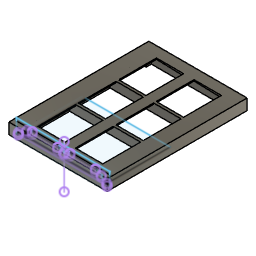
case_basic_v1 (Autodesk Fusion 360 archive; units mm, degrees)
design "lid fitting"
Autodesk Fusion 360 part; units mm, degrees
sketch "Skizze1" plane through (0, 0, 0) normal (0, 1, 0) x (1, 0, 0)
  line L0 (0, 0) -> (66.84, 0)
  line L1 (66.84, 0) -> (66.84, -1.6)
  line L2 (66.84, -1.6) -> (0, -1.6)
  line L3 (0, -1.6) -> (0, 0)
  line L4 (6.12, -13) -> (6.12, 20) construction
  line L5 (6.12, -4.35) -> (34.0577, -3.52)
  line L6 (6.1556, -5.5495) -> (34.0933, -4.7195)
  line L7 (34.0933, -4.7195) -> (34.0577, -3.52)
  line L8 (6.1556, -5.5495) -> (6.12, -4.35)
  line L9 (10.5057, -7.171) -> (29.6972, -6.6008)
  line L10 (10.5057, -7.171) -> (10.4537, -5.4218)
  line L11 (29.6972, -6.6008) -> (29.6453, -4.8516)
  line L12 (34.6056, -5.5495) -> (62.5433, -4.7195)
  line L13 (34.57, -13) -> (34.57, 20) construction
  line L14 (38.9557, -7.171) -> (38.9037, -5.4218)
  line L15 (34.57, -4.35) -> (62.5077, -3.52)
  line L16 (34.6056, -5.5495) -> (34.57, -4.35)
  line L17 (38.9557, -7.171) -> (58.1472, -6.6008)
  line L18 (62.5433, -4.7195) -> (62.5077, -3.52)
  line L19 (58.1472, -6.6008) -> (58.0953, -4.8516)
  dimension "d1" = 66.84
  dimension "d2" = 1.6
  dimension "d3" = 6.12
  dimension "d4" = 2.75
  dimension "d5" = 1.92
  dimension "d6" = 27.95
  dimension "d7" = 1.2
  dimension "d8" = 1.75
  dimension "d9" = 4.3
  dimension "d10" = 19.2
  dimension "d11" = 1.2
  dimension "d12" = 27.95
  dimension "d13" = 1.75
  dimension "d14" = 4.3
  dimension "d15" = 19.2
  constraint horizontal L0
  constraint vertical L1
  constraint horizontal L2
  constraint vertical L3
  constraint coincident L0.start L3.end
  constraint perpendicular L0 L4
  constraint coincident L4 L5.start
  constraint perpendicular L5 L7
  constraint perpendicular L5 L8
  constraint parallel L6 L9
  constraint coincident L6 L10.end
  constraint perpendicular L6 L10
  constraint coincident L6 L11.end
  constraint perpendicular L6 L11
  constraint coincident L15.start L13
  constraint perpendicular L15 L18
  constraint perpendicular L15 L16
  constraint parallel L12 L17
  constraint coincident L14.end L12
  constraint perpendicular L12 L14
  constraint coincident L19.end L12
  constraint perpendicular L12 L19
  measures "d1" distance of L0.start L0.end
  measures "d2" distance of L0.start L2.end
  measures "d3" distance of L3 L4
  measures "d4" distance of L2 L5.start
  measures "d5" distance of L2 L5.end
  measures "d6" distance of L5.start L5.end
  measures "d8" distance of L6 L9
  measures "d9" distance of L8 L10
  measures "d10" distance of L10 L11
  measures "d12" distance of L15.end L15.start
  measures "d13" distance of L12 L17
  measures "d14" distance of L14 L16
  measures "d15" distance of L14 L19
sketch "Skizze2" plane through (0, 0, 0) normal (0, 1, 0) x (1, 0, 0)
  line L0 (0, -1.65) -> (5.6396, -1.65)
  line L1 (5.6396, -1.65) -> (5.8137, -7.5105)
  line L2 (5.8137, -7.5105) -> (30.6972, -6.7712)
  line L3 (34.5575, -5.9701) -> (34.6029, -7.5004)
  line L4 (34.6029, -7.5004) -> (59.1472, -6.7712)
  line L5 (63.4939, -1.65) -> (67.24, -1.65)
  line L6 (67.24, -1.65) -> (67.24, 0)
  line L7 (0, -1.65) -> (-0.4, -1.65)
  line L8 (-0.4, -1.65) -> (-0.4, 0)
  line L9 (-0.4, 0) -> (-1.5, 0)
  line L10 (-1.5, 0) -> (-1.5, -10.4859)
  line L11 (-1.5, -10.4859) -> (69, -10.4859)
  line L12 (69, -10.4859) -> (69, 0)
  line L13 (69, 0) -> (67.24, 0)
  line L14 (10.5057, -7.171) -> (29.6972, -6.6008)
  line L15 (38.9557, -7.171) -> (58.1472, -6.6008)
  line L16 (38.9557, -7.171) -> (38.9037, -5.4218)
  line L17 (34.6056, -5.5495) -> (62.5433, -4.7195)
  line L18 (34.6056, -5.5495) -> (34.57, -4.35)
  line L19 (6.1556, -5.5495) -> (34.0933, -4.7195)
  line L20 (29.6972, -6.6008) -> (29.6453, -4.8516)
  line L21 (6.1556, -5.5495) -> (6.12, -4.35)
  line L22 (62.5433, -4.7195) -> (62.5077, -3.52)
  line L23 (58.1472, -6.6008) -> (58.0953, -4.8516)
  line L24 (0, -1.6) -> (0, 0)
  line L25 (66.84, -1.6) -> (0, -1.6)
  line L26 (10.5057, -7.171) -> (10.4537, -5.4218)
  line L27 (66.84, 0) -> (66.84, -1.6)
  line L28 (59.1472, -6.7712) -> (63.3193, -5.3134)
  line L29 (30.6972, -6.7712) -> (34.5575, -5.9701)
  line L30 (34.6029, -7.5004) -> (30.6972, -8.2712)
  line L31 (30.6972, -8.2712) -> (30.6972, -6.7712)
  line L32 (34.57, -13) -> (34.57, 20)
  line L33 (59.1472, -6.7712) -> (59.1472, -8.2712)
  line L34 (59.1472, -8.2712) -> (69, -8.2712)
  line L35 (30.6972, -8.2712) -> (38.5, -8.2712)
  line L36 (38.5, -8.2712) -> (38.5, -7.3846)
  line L37 (10.1496, -8.2712) -> (10.1496, -7.3817)
  line L38 (10.1496, -8.2712) -> (6, -8.2712)
  line L39 (6, -8.2712) -> (-1.5, -8.2712)
  line L40 (10.1496, -8.2712) -> (30.6972, -8.2712)
  line L41 (38.5, -8.2712) -> (59.1472, -8.2712)
  line L42 (0, 0) -> (66.84, 0)
  line L43 (-0.4, -1.65) -> (67.24, -1.65)
  line L44 (-0.4, 0) -> (67.24, 0)
  line L45 (63.3193, -5.3134) -> (63.4939, -1.65)
  dimension "d16" = 0.4
  dimension "d17" = 0.05
  dimension "d18" = 0.4
  dimension "d21" = 0.2
  dimension "d27" = 0.2
  dimension "d32" = 0.05
  dimension "d33" = 0.4
  dimension "d39" = 1
  dimension "d40" = 1.5
  dimension "d41" = 1
  dimension "d42" = 1.5
  constraint horizontal L0
  constraint horizontal L5
  constraint parallel L0 L7
  constraint perpendicular L8 L9
  constraint perpendicular L9 L10
  constraint perpendicular L10 L11
  constraint perpendicular L11 L12
  constraint perpendicular L6 L13
  constraint parallel L2 L14
  constraint parallel L4 L15
  constraint parallel L3 L16
  constraint parallel L1 L21
  constraint parallel L31 L32
  constraint vertical L33
  constraint coincident L12 L34.end
  constraint perpendicular L12 L34
  constraint perpendicular L31 L35
  constraint coincident L4 L36.end
  constraint perpendicular L35 L36
  constraint coincident L2 L37.end
  constraint parallel L31 L37
  constraint perpendicular L37 L38
  constraint coincident L10 L39.end
  constraint perpendicular L10 L39
  constraint perpendicular L31 L40
  constraint collinear L9 L42
  constraint collinear L13 L42
  constraint coincident L8 L9.start
  constraint coincident L6 L13.end
  constraint perpendicular L6 L44
  constraint collinear L9 L44
  measures "d16" distance of L8 L24
  measures "d17" distance of L0 L25
  measures "d18" distance of L1 L21
  measures "d21" distance of L2 L14
  measures "d27" distance of L4 L15
  measures "d32" distance of L5 L25
  measures "d33" distance of L6 L27
  measures "d39" distance of L14.end L31
  measures "d40" distance of L2.end L30.end
  measures "d41" distance of L15.end L33
  measures "d42" distance of L4.end L33.end
extrude "Extrusion2" add sketch "Skizze1" sketch "Skizze2" against normal blind 3.5 contours L0 L1 L2 L3 | L6 L9 L10 L11 | L12 L14 L17 L19 of sketch 2 contours L0 L7 L8 L24 L25 L32 L43 L44 | L0 L1 L2 L7 L8 L9 L10 L37 L38 L39 L43 | L1 L2 L3 L29 L32 L43 | L3 L4 L28 L32 L43 L45 | L5 L6 L25 L27 L32 L43 L44 | L2 L31 L37 L40 | L5 L6 L12 L13 L28 L33 L34 L43 L45 | L3 L29 L30 L31 L32 | L30 L32 L35 | L4 L30 L32 L35 L36 | L4 L33 L36 L41
extrude "Extrusion1" add sketch "Skizze2" along normal blind 4.6 contours L0 L1 L2 L7 L8 L9 L10 L37 L38 L39 L43 | L2 L31 L37 L40 | L5 L6 L12 L13 L28 L33 L34 L43 L45 | L3 L29 L30 L31 L32 | L3 L30 L32 | L30 L32 L35 | L4 L30 L32 L35 L36 | L4 L33 L36 L41
extrude "Extrusion3" add sketch "Skizze2" along normal blind 28.5 from surface at 4.6 contours L0 L1 L2 L7 L8 L9 L10 L37 L38 L39 L43 | L5 L6 L12 L13 L28 L33 L34 L43 L45 | L3 L29 L30 L31 L32 | L30 L32 L35 | L4 L30 L32 L35 L36
extrude "Extrusion4" add sketch "Skizze2" along normal blind 2 from surface at 33.1 contours L0 L1 L2 L7 L8 L9 L10 L37 L38 L39 L43 | L1 L2 L3 L29 L32 L43 | L3 L4 L28 L32 L43 L45 | L2 L31 L37 L40 | L5 L6 L12 L13 L28 L33 L34 L43 L45 | L3 L29 L30 L31 L32 | L30 L32 L35 | L4 L30 L32 L35 L36 | L4 L33 L36 L41 | L14 L19 L20 L26 | L15 L16 L17 L23
extrude "Extrusion5" add sketch "Skizze2" along normal blind 14.25 from surface at 35.1 contours L0 L1 L2 L7 L8 L9 L10 L37 L38 L39 L43 | L5 L6 L12 L13 L28 L33 L34 L43 L45 | L3 L29 L30 L31 L32 | L30 L32 L35 | L4 L30 L32 L35 L36
extrude "Extrusion10" add sketch "Skizze2" along normal blind 3.9 contours L1 L2 L3 L29 L32 L43 | L3 L4 L28 L32 L43 L45 | L14 L19 L20 L26 | L15 L16 L17 L23
sketch "Skizze4" plane through (0, 0, 0) normal (0, 0, -1) x (1, 0, 0)
  line L0 (-0.4, 0) -> (67.24, 0)
  line L1 (67.24, 0) -> (67.24, -49.35)
  line L2 (67.24, -49.35) -> (69, -49.35)
  line L3 (69, -49.35) -> (69, 3.5)
  line L4 (69, 3.5) -> (-1.5, 3.5)
  line L5 (-1.5, 3.5) -> (-1.5, -49.35)
  line L6 (-1.5, -49.35) -> (-0.4, -49.35)
  line L7 (-0.4, -49.35) -> (-0.4, 0)
  line L8 (65.24, -49.35) -> (1.6, -49.35)
  line L9 (1.6, -49.35) -> (1.6, -2)
  line L10 (1.6, -2) -> (65.24, -2)
  line L11 (65.24, -2) -> (65.24, -49.35)
  line L12 (-0.4, 0) -> (67.24, 0)
  circle A0 centre (63.74, -3.5) radius 1.5 construction
  circle A1 centre (3.1, -3.5) radius 1.5 construction
  circle A2 centre (63.74, -3.5) radius 1.45
  circle A3 centre (3.1, -3.5) radius 1.45
  dimension "d62" = 2
  dimension "d63" = 2
  dimension "d64" = 2
  dimension "d65" = 1.5
  dimension "d66" = 1.5
  dimension "d67" = -0.05
  dimension "d68" = -0.05
  constraint horizontal L8
  constraint vertical L9
  constraint horizontal L10
  constraint vertical L11
  constraint tangent L11 A0
  constraint tangent L10 A0
  constraint tangent L10 A1
  constraint tangent L9 A1
  measures "d62" distance of L1 L11
  measures "d63" distance of L7 L9
  measures "d64" distance of L10 L12
  measures "d65" radius of A0
  measures "d66" radius of A1
extrude "Extrusion7" cut sketch "Skizze4" against normal blind 6 contours A2 | A3
mirror "Spiegeln1" about plane through (0, 49.35, 0) normal (0, 1, 0) of bodies 1 merged
sketch "Skizze5" plane through (0, 0, 1.65) normal (0, 0, -1) x (1, 0, 0)
  line L0 (5.6396, -63.6) -> (5.6396, -35.1)
  line L1 (5.6396, -35.1) -> (63.4939, -35.1)
  line L2 (63.4939, -63.6) -> (5.6396, -63.6)
  line L3 (-0.4, 0) -> (-0.4, -98.7)
  line L4 (-0.4, -98.7) -> (67.24, -98.7)
  line L5 (5.6396, -94.8) -> (5.6396, -65.6)
  line L6 (5.6396, -65.6) -> (63.4939, -65.6)
  arc A0 (62.3463, -94.8) -> (63.4939, -93.771) centre (63.74, -95.2) ccw
  line L7 (67.24, -98.7) -> (67.24, 0)
  arc A1 (63.4939, -4.929) -> (62.3463, -3.9) centre (63.74, -3.5) ccw
  line L8 (63.4939, -33.1) -> (5.6396, -33.1)
  line L9 (5.6396, -33.1) -> (5.6396, -3.9)
  line L10 (67.24, 0) -> (-0.4, 0)
  line L11 (-0.4, -90.85) -> (6.6, -90.85)
  line L12 (6.6, -90.85) -> (6.6, -68.85)
  line L13 (6.6, -68.85) -> (-0.4, -68.85)
  line L14 (-0.4, -68.85) -> (-0.4, -90.85)
  line L15 (-0.4, 0) -> (-0.4, -98.7)
  line L16 (30.6972, -94.1) -> (30.6972, -65.6)
  line L17 (30.6972, -79.85) -> (-17.4972, -79.85)
  line L18 (63.4939, -35.1) -> (63.4939, -63.6)
  line L19 (63.4939, -65.6) -> (63.4939, -93.771)
  line L20 (63.4939, -4.929) -> (63.4939, -33.1)
  circle A2 centre (3.1, -95.2) radius 1.45
  circle A3 centre (3.1, -3.5) radius 1.45
  line L21 (-0.4, -98.7) -> (67.24, -98.7)
  line L22 (62.3463, -94.8) -> (5.6396, -94.8)
  line L23 (5.6396, -3.9) -> (62.3463, -3.9)
  dimension "d80" = 7
  dimension "d81" = 22
  constraint horizontal L11
  constraint vertical L14
  constraint coincident L3 L11.start
  constraint parallel L12 L15
  constraint midpoint L16 L17.start
  constraint perpendicular L5 L17
  constraint midpoint L12 L17
  measures "d80" distance of L12 L15
  measures "d81" distance of L11 L13
extrude "Extrusion9" cut sketch "Skizze5" against normal blind 3 contours L3 L5 L13 L14 L15 L17 | L3 L5 L11 L14 L15 L17 | L5 L12 L13 L17 | L5 L11 L12 L17
move_face "Flächen versetzen1" offset 1.54 1 faces at (69, 66.9667, 5.5141)
move_face "Flächen versetzen2" offset 2.2 1 faces at (-1.5, 66.9667, 2.7571)
